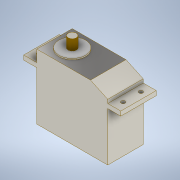
# Autodesk Inventor part: big_servo
Saved by Autodesk Inventor 2020.3 (Build 243373000, 373)
## iProperties
Created: 2020-08-06
Part Number: big_servo
Material: PPS Plastic
Document SubType Name: Modeling
Designer: aditk
Density: 1.637 g/cm^3
Appearance: Titanium - Polished
Author: aditk
Autodesk Inventor part; units mm, degrees
ref_plane "YZ Plane" through (0, 0, 0) normal (1, 0, 0) x (0, 1, 0)
ref_plane "XZ Plane" through (0, 0, 0) normal (0, 1, 0) x (-1, 0, 0)
ref_plane "XY Plane" through (0, 0, 0) normal (0, 0, 1) x (1, 0, 0)
sketch "Sketch1" plane through (0, 0, 0) normal (0, 1, 0) x (-1, 0, 0)
  line L0 (20.1, -10.05) -> (-20.1, -10.05)
  line L1 (-20.1, -10.05) -> (-20.1, 10.05)
  line L2 (-20.1, 10.05) -> (20.1, 10.05)
  line L3 (20.1, 10.05) -> (20.1, -10.05)
  line L4 (20.1, -10.05) -> (-20.1, 10.05) construction
  line L5 (-20.1, -10.05) -> (20.1, 10.05) construction
  point P0 (0, 0)
  dimension "d0" = 40.2
  dimension "d1" = 20.1
  constraints: 12 end point, 2 midpoint, 2 parallel, 1 horizontal, 1 perpendicular
  measures "d0" distance of L1.end L2.end
  measures "d1" distance of L0.end L1.end
extrude "Extrusion1" add sketch "Sketch1" along normal blind 27.7
sketch "Sketch2" plane through (0, 27.7, 0) normal (0, 1, 0) x (1, 0, 0)
  line L0 (27.5, -10.05) -> (-27.5, -10.05)
  line L1 (-27.5, -10.05) -> (-27.5, 10.05)
  line L2 (-27.5, 10.05) -> (27.5, 10.05)
  line L3 (27.5, 10.05) -> (27.5, -10.05)
  line L4 (27.5, -10.05) -> (-27.5, 10.05) construction
  line L5 (-27.5, -10.05) -> (27.5, 10.05) construction
  point P0 (0, 0)
  dimension "d4" = 55
  constraints: 12 end point, 2 midpoint, 2 parallel, 1 horizontal, 1 perpendicular
  measures "d4" distance of L1.end L2.end
extrude "Extrusion2" add sketch "Sketch2" along normal blind 2.5
sketch "Sketch3" plane through (0, 30.2, 0) normal (0, 1, 0) x (1, 0, 0)
  line L0 (-27.5, -10.05) -> (27.5, -10.05) projected
  line L1 (-20.1, 10.05) -> (20.1, 10.05) projected
  line L2 (20.1, 10.05) -> (20.1, -10.05) projected
  line L3 (20.1, -10.05) -> (-20.1, -10.05) projected
  line L4 (-20.1, -10.05) -> (-20.1, 10.05) projected
  line L5 (27.5, 10.05) -> (-27.5, 10.05) projected
  line L6 (-27.5, 10.05) -> (-27.5, -10.05) projected
  line L7 (27.5, -10.05) -> (27.5, 10.05) projected
  line L8 (20.1, 10.05) -> (20.1, -10.05) projected
  line L9 (27.5, 10.05) -> (27.5, -10.05) projected
  circle A0 centre (23.8, 5.025) radius 1.1
  line L10 (20.1, -10.05) -> (-20.1, -10.05) projected
  line L11 (-20.1, 10.05) -> (20.1, 10.05) projected
  circle A1 centre (-23.8, 5.025) radius 1.1
  circle A2 centre (23.8, -5.025) radius 1.1
  circle A3 centre (-23.8, -5.025) radius 1.1
  point P0 (0, 0)
  constraints: 4 centre point
extrude "Extrusion3" cut sketch "Sketch3" against normal through all contours A0 | A1 | A2 | A3
sketch "Sketch4" plane through (20.1, 0, -10.05) normal (0, 0, -1) x (-1, 0, 0)
  line L0 (0, 0) -> (0, 36.8)
  line L1 (0, 36.8) -> (40.2, 36.8)
  line L2 (40.2, 0) -> (40.2, 27.7) projected
  line L3 (40.2, 36.8) -> (40.2, 0)
  line L4 (40.2, 0) -> (0, 0)
  line L5 (-7.4, 30.2) -> (47.6, 30.2) projected
  line L6 (0, 30.2) -> (40.2, 30.2)
  point P0 (20.1, 0)
  dimension "d10" = 36.8
  constraints: 10 end point, 4 point on line, 2 perpendicular, 1 collinear, 1 vertical
  measures "d10" distance of L0.start L0.end
extrude "Extrusion4" add sketch "Sketch4" against normal up to surface (20.1 mm away) contours L0 L1 L3 L5
sketch "Sketch5" plane through (-20.1, 36.8, -10.05) normal (0, 1, 0) x (1, 0, 0)
  line L0 (20.1, -10.05) -> (0, -10.05)
  line L1 (10.05, -10.05) -> (10.05, 0)
  line L2 (0, 0) -> (40.2, 0) projected
  circle A0 centre (10.05, -10.05) radius 7.5
  dimension "d13" = 15
  constraints: 4 end point, 1 centre point, 1 coincident, 1 horizontal, 1 midpoint, 1 point on line, 1 vertical
  measures "d13" diameter of A0
extrude "Extrusion5" add sketch "Sketch5" along normal blind 0.7
sketch "Sketch6" plane through (-10.05, 37.5, 0) normal (0, 1, 0) x (1, 0, 0)
  circle A0 centre (0, 0) radius 2.25
  point P0 (10.05, 0)
  dimension "d16" = 4.5
  constraints: 1 centre point
  measures "d16" diameter of A0
extrude "Extrusion6" add sketch "Sketch6" along normal blind 6
chamfer "Chamfer1" distance 9.75 angle 25 1 edges at (20.1, 36.8, 0) measured on face at (12.55, 36.8, 0)
sketch "Sketch7" plane through (-10.05, 43.5, 0) normal (0, 1, 0) x (1, 0, 0)
  line L0 (0, 0) -> (0, -2.25)
  circle A0 centre (0, 0) radius 2.25 projected
  line L1 (0, -2.25) -> (0, -2.35)
  line L2 (0, -2.35) -> (0.1023, -2.2477)
  line L3 (0, -2.35) -> (-0.1023, -2.2477)
  point P0 (10.05, 0)
  point P1 (-0.1023, -2.2477)
  dimension "d22" = 0.1
  dimension "d23" = 45
  constraints: 8 end point, 2 point on circle, 1 point on line, 1 symmetric about line, 1 vertical
  measures "d22" distance of L0.end L1.end
  measures "d23" angle of L2 L1
extrude "Extrusion7" add sketch "Sketch7" against normal up to surface (6 mm away) contours A0 L1 L3 | L2 L1 A0
pattern_circular "Circular Pattern1" count 80 over 360 about axis through (-10.05, 37.5, 0) along (0, 1, 0) of "Extrusion7"
sketch "Sketch8" plane through (-20.1, 36.8, 10.05) normal (0, 1, 0) x (1, 0, 0)
  line L0 (40.2, 20.1) -> (40.2, 0) projected
  line L1 (40.2, 0) -> (47.6, 0) projected
  line L2 (47.6, 0) -> (47.6, 20.1) projected
  line L3 (47.6, 20.1) -> (40.2, 20.1) projected
  circle A0 centre (43.9, 5.025) radius 1.1 projected
  circle A1 centre (43.9, 15.075) radius 1.1 projected
  line L4 (30.45, 0) -> (40.2, 0) projected
  line L5 (40.2, 0) -> (40.2, 20.1) projected
  line L6 (40.2, 20.1) -> (30.45, 20.1) projected
  line L7 (30.45, 20.1) -> (30.45, 0) projected
  line L8 (30.45, 20.1) -> (30.45, 0) projected
  line L9 (0, 20.1) -> (30.45, 20.1) projected
  line L10 (0, 20.1) -> (0, 0) projected
  line L11 (0, 0) -> (30.45, 0) projected
  circle A2 centre (10.05, 10.05) radius 7.5 projected
  line L12 (0, 0) -> (0, 20.1) projected
  line L13 (0, 20.1) -> (-7.4, 20.1) projected
  line L14 (-7.4, 20.1) -> (-7.4, 0) projected
  line L15 (-7.4, 0) -> (0, 0) projected
  circle A3 centre (-3.7, 5.025) radius 1.1 projected
  circle A4 centre (-3.7, 15.075) radius 1.1 projected
  circle A5 centre (10.05, 10.05) radius 7.5 projected
  line L16 (9.9612, 7.7888) -> (9.8656, 7.7072) projected
  line L17 (9.8656, 7.7072) -> (9.784, 7.8028) projected
  line L18 (9.784, 7.8028) -> (9.6824, 7.7289) projected
  line L19 (9.6824, 7.7289) -> (9.6085, 7.8306) projected
  line L20 (9.6085, 7.8306) -> (9.5014, 7.7649) projected
  line L21 (9.5014, 7.7649) -> (9.4358, 7.8721) projected
  line L22 (9.4358, 7.8721) -> (9.3238, 7.815) projected
  line L23 (9.3238, 7.815) -> (9.2668, 7.927) projected
  line L24 (9.2668, 7.927) -> (9.1507, 7.8789) projected
  line L25 (9.1507, 7.8789) -> (9.1026, 7.995) projected
  line L26 (9.1026, 7.995) -> (8.9831, 7.9561) projected
  line L27 (8.9831, 7.9561) -> (8.9443, 8.0756) projected
  line L28 (8.9443, 8.0756) -> (8.8221, 8.0463) projected
  line L29 (8.8221, 8.0463) -> (8.7928, 8.1685) projected
  line L30 (8.7928, 8.1685) -> (8.6687, 8.1488) projected
  line L31 (8.6687, 8.1488) -> (8.6491, 8.2729) projected
  line L32 (8.6491, 8.2729) -> (8.5238, 8.263) projected
  line L33 (8.5238, 8.263) -> (8.5139, 8.3883) projected
  line L34 (8.5139, 8.3883) -> (8.3883, 8.3883) projected
  line L35 (8.3883, 8.3883) -> (8.3883, 8.5139) projected
  line L36 (8.3883, 8.5139) -> (8.263, 8.5238) projected
  line L37 (8.263, 8.5238) -> (8.2729, 8.6491) projected
  line L38 (8.2729, 8.6491) -> (8.1488, 8.6687) projected
  line L39 (8.1488, 8.6687) -> (8.1685, 8.7928) projected
  line L40 (8.1685, 8.7928) -> (8.0463, 8.8221) projected
  line L41 (8.0463, 8.8221) -> (8.0756, 8.9443) projected
  line L42 (8.0756, 8.9443) -> (7.9561, 8.9831) projected
  line L43 (7.9561, 8.9831) -> (7.995, 9.1026) projected
  line L44 (7.995, 9.1026) -> (7.8789, 9.1507) projected
  line L45 (7.8789, 9.1507) -> (7.927, 9.2668) projected
  line L46 (7.927, 9.2668) -> (7.815, 9.3238) projected
  line L47 (7.815, 9.3238) -> (7.8721, 9.4358) projected
  line L48 (7.8721, 9.4358) -> (7.7649, 9.5014) projected
  line L49 (7.7649, 9.5014) -> (7.8306, 9.6085) projected
  line L50 (7.8306, 9.6085) -> (7.7289, 9.6824) projected
  line L51 (7.7289, 9.6824) -> (7.8028, 9.784) projected
  line L52 (7.8028, 9.784) -> (7.7072, 9.8656) projected
  line L53 (7.7072, 9.8656) -> (7.7888, 9.9612) projected
  line L54 (7.7888, 9.9612) -> (7.7, 10.05) projected
  line L55 (7.7, 10.05) -> (7.7888, 10.1388) projected
  line L56 (7.7888, 10.1388) -> (7.7072, 10.2344) projected
  line L57 (7.7072, 10.2344) -> (7.8028, 10.316) projected
  line L58 (7.8028, 10.316) -> (7.7289, 10.4176) projected
  line L59 (7.7289, 10.4176) -> (7.8306, 10.4915) projected
  line L60 (7.8306, 10.4915) -> (7.7649, 10.5986) projected
  line L61 (7.7649, 10.5986) -> (7.8721, 10.6642) projected
  line L62 (7.8721, 10.6642) -> (7.815, 10.7762) projected
  line L63 (7.815, 10.7762) -> (7.927, 10.8332) projected
  line L64 (7.927, 10.8332) -> (7.8789, 10.9493) projected
  line L65 (7.8789, 10.9493) -> (7.995, 10.9974) projected
  line L66 (7.995, 10.9974) -> (7.9561, 11.1169) projected
  line L67 (7.9561, 11.1169) -> (8.0756, 11.1557) projected
  line L68 (8.0756, 11.1557) -> (8.0463, 11.2779) projected
  line L69 (8.0463, 11.2779) -> (8.1685, 11.3072) projected
  line L70 (8.1685, 11.3072) -> (8.1488, 11.4313) projected
  line L71 (8.1488, 11.4313) -> (8.2729, 11.4509) projected
  line L72 (8.2729, 11.4509) -> (8.263, 11.5762) projected
  line L73 (8.263, 11.5762) -> (8.3883, 11.5861) projected
  line L74 (8.3883, 11.5861) -> (8.3883, 11.7117) projected
  line L75 (8.3883, 11.7117) -> (8.5139, 11.7117) projected
  line L76 (8.5139, 11.7117) -> (8.5238, 11.837) projected
  line L77 (8.5238, 11.837) -> (8.6491, 11.8271) projected
  line L78 (8.6491, 11.8271) -> (8.6687, 11.9512) projected
  line L79 (8.6687, 11.9512) -> (8.7928, 11.9315) projected
  line L80 (8.7928, 11.9315) -> (8.8221, 12.0537) projected
  line L81 (8.8221, 12.0537) -> (8.9443, 12.0244) projected
  line L82 (8.9443, 12.0244) -> (8.9831, 12.1439) projected
  line L83 (8.9831, 12.1439) -> (9.1026, 12.105) projected
  line L84 (9.1026, 12.105) -> (9.1507, 12.2211) projected
  line L85 (9.1507, 12.2211) -> (9.2668, 12.173) projected
  line L86 (9.2668, 12.173) -> (9.3238, 12.285) projected
  line L87 (9.3238, 12.285) -> (9.4358, 12.2279) projected
  line L88 (9.4358, 12.2279) -> (9.5014, 12.3351) projected
  line L89 (9.5014, 12.3351) -> (9.6085, 12.2694) projected
  line L90 (9.6085, 12.2694) -> (9.6824, 12.3711) projected
  line L91 (9.6824, 12.3711) -> (9.784, 12.2972) projected
  line L92 (9.784, 12.2972) -> (9.8656, 12.3928) projected
  line L93 (9.8656, 12.3928) -> (9.9612, 12.3112) projected
  line L94 (9.9612, 12.3112) -> (10.05, 12.4) projected
  line L95 (10.05, 12.4) -> (10.1388, 12.3112) projected
  line L96 (10.1388, 12.3112) -> (10.2344, 12.3928) projected
  line L97 (10.2344, 12.3928) -> (10.316, 12.2972) projected
  line L98 (10.316, 12.2972) -> (10.4176, 12.3711) projected
  line L99 (10.4176, 12.3711) -> (10.4915, 12.2694) projected
  line L100 (10.4915, 12.2694) -> (10.5986, 12.3351) projected
  line L101 (10.5986, 12.3351) -> (10.6642, 12.2279) projected
  line L102 (10.6642, 12.2279) -> (10.7762, 12.285) projected
  line L103 (10.7762, 12.285) -> (10.8332, 12.173) projected
  line L104 (10.8332, 12.173) -> (10.9493, 12.2211) projected
  line L105 (10.9493, 12.2211) -> (10.9974, 12.105) projected
  line L106 (10.9974, 12.105) -> (11.1169, 12.1439) projected
  line L107 (11.1169, 12.1439) -> (11.1557, 12.0244) projected
  line L108 (11.1557, 12.0244) -> (11.2779, 12.0537) projected
  line L109 (11.2779, 12.0537) -> (11.3072, 11.9315) projected
  line L110 (11.3072, 11.9315) -> (11.4313, 11.9512) projected
  line L111 (11.4313, 11.9512) -> (11.4509, 11.8271) projected
  line L112 (11.4509, 11.8271) -> (11.5762, 11.837) projected
  line L113 (11.5762, 11.837) -> (11.5861, 11.7117) projected
  line L114 (11.5861, 11.7117) -> (11.7117, 11.7117) projected
  line L115 (11.7117, 11.7117) -> (11.7117, 11.5861) projected
  line L116 (11.7117, 11.5861) -> (11.837, 11.5762) projected
  line L117 (11.837, 11.5762) -> (11.8271, 11.4509) projected
  line L118 (11.8271, 11.4509) -> (11.9512, 11.4313) projected
  line L119 (11.9512, 11.4313) -> (11.9315, 11.3072) projected
  line L120 (11.9315, 11.3072) -> (12.0537, 11.2779) projected
  line L121 (12.0537, 11.2779) -> (12.0244, 11.1557) projected
  line L122 (12.0244, 11.1557) -> (12.1439, 11.1169) projected
  line L123 (12.1439, 11.1169) -> (12.105, 10.9974) projected
  line L124 (12.105, 10.9974) -> (12.2211, 10.9493) projected
  line L125 (12.2211, 10.9493) -> (12.173, 10.8332) projected
  line L126 (12.173, 10.8332) -> (12.285, 10.7762) projected
  line L127 (12.285, 10.7762) -> (12.2279, 10.6642) projected
  line L128 (12.2279, 10.6642) -> (12.3351, 10.5986) projected
  line L129 (12.3351, 10.5986) -> (12.2694, 10.4915) projected
  line L130 (12.2694, 10.4915) -> (12.3711, 10.4176) projected
  line L131 (12.3711, 10.4176) -> (12.2972, 10.316) projected
  line L132 (12.2972, 10.316) -> (12.3928, 10.2344) projected
  line L133 (12.3928, 10.2344) -> (12.3112, 10.1388) projected
  line L134 (12.3112, 10.1388) -> (12.4, 10.05) projected
  line L135 (12.4, 10.05) -> (12.3112, 9.9612) projected
  line L136 (12.3112, 9.9612) -> (12.3928, 9.8656) projected
  line L137 (12.3928, 9.8656) -> (12.2972, 9.784) projected
  line L138 (12.2972, 9.784) -> (12.3711, 9.6824) projected
  line L139 (12.3711, 9.6824) -> (12.2694, 9.6085) projected
  line L140 (12.2694, 9.6085) -> (12.3351, 9.5014) projected
  line L141 (12.3351, 9.5014) -> (12.2279, 9.4358) projected
  line L142 (12.2279, 9.4358) -> (12.285, 9.3238) projected
  line L143 (12.285, 9.3238) -> (12.173, 9.2668) projected
  line L144 (12.173, 9.2668) -> (12.2211, 9.1507) projected
  line L145 (12.2211, 9.1507) -> (12.105, 9.1026) projected
  line L146 (12.105, 9.1026) -> (12.1439, 8.9831) projected
  line L147 (12.1439, 8.9831) -> (12.0244, 8.9443) projected
  line L148 (12.0244, 8.9443) -> (12.0537, 8.8221) projected
  line L149 (12.0537, 8.8221) -> (11.9315, 8.7928) projected
  line L150 (11.9315, 8.7928) -> (11.9512, 8.6687) projected
  line L151 (11.9512, 8.6687) -> (11.8271, 8.6491) projected
  line L152 (11.8271, 8.6491) -> (11.837, 8.5238) projected
  line L153 (11.837, 8.5238) -> (11.7117, 8.5139) projected
  line L154 (11.7117, 8.5139) -> (11.7117, 8.3883) projected
  line L155 (11.7117, 8.3883) -> (11.5861, 8.3883) projected
  line L156 (11.5861, 8.3883) -> (11.5762, 8.263) projected
  line L157 (11.5762, 8.263) -> (11.4509, 8.2729) projected
  line L158 (11.4509, 8.2729) -> (11.4313, 8.1488) projected
  line L159 (11.4313, 8.1488) -> (11.3072, 8.1685) projected
  line L160 (11.3072, 8.1685) -> (11.2779, 8.0463) projected
  line L161 (11.2779, 8.0463) -> (11.1557, 8.0756) projected
  line L162 (11.1557, 8.0756) -> (11.1169, 7.9561) projected
  line L163 (11.1169, 7.9561) -> (10.9974, 7.995) projected
  line L164 (10.9974, 7.995) -> (10.9493, 7.8789) projected
  line L165 (10.9493, 7.8789) -> (10.8332, 7.927) projected
  line L166 (10.8332, 7.927) -> (10.7762, 7.815) projected
  line L167 (10.7762, 7.815) -> (10.6642, 7.8721) projected
  line L168 (10.6642, 7.8721) -> (10.5986, 7.7649) projected
  line L169 (10.5986, 7.7649) -> (10.4915, 7.8306) projected
  line L170 (10.4915, 7.8306) -> (10.4176, 7.7289) projected
  line L171 (10.4176, 7.7289) -> (10.316, 7.8028) projected
  line L172 (10.316, 7.8028) -> (10.2344, 7.7072) projected
  line L173 (10.2344, 7.7072) -> (10.1388, 7.7888) projected
  line L174 (10.1388, 7.7888) -> (10.05, 7.7) projected
  line L175 (10.05, 7.7) -> (9.9612, 7.7888) projected
  point P0 (20.1, 10.05)
body "Solid1"
